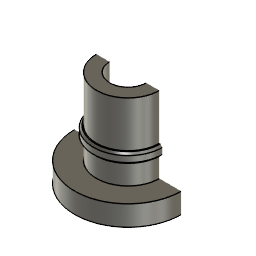
Alfa 147 Handle Saddle V3 - 3.6mm (Autodesk Fusion 360 design; units mm, degrees)
Autodesk Fusion 360 part; units mm, degrees
sketch "Sketch1" plane through (0, 0, 0) normal (0, 0, 1) x (1, 0, 0)
  circle A0 centre (0, 0) radius 5.25
  circle A1 centre (0, 0) radius 3.1
  circle A2 centre (0, 0) radius 1.8
  circle A3 centre (0, 0) radius 3.4
  circle A4 centre (0, 0) radius 1.5
  dimension "d1" = 10.5
  dimension "d2" = 6.2
  dimension "d3" = 3.6
  dimension "d21" = 0.3
  dimension "d22" = 0.3
  constraint coincident A0.centre A1.centre
  constraint concentric A0 A2
  constraint concentric A2 A3
  constraint concentric A1 A4
  measures "d1" diameter of A0
  measures "d2" diameter of A1
  measures "d3" diameter of A2
  measures "d21" distance of A2 A4
  measures "d22" distance of A1 A3
extrude "Extrude1" add sketch "Sketch1" along normal blind 9.5 contours A1
extrude "Extrude2" add sketch "Sketch1" along normal blind 2 contours A0 | A3
extrude "Extrude3" add sketch "Sketch1" along normal blind 4 and the other way blind -5 contours A3
chamfer "Chamfer1" distance 0.2 angle 45 2 edges at (-3.1699, -1.2295, 4) (-3.1699, -1.2295, 5)
chamfer "Chamfer2" distance 0.5 angle 45 1 edges at (-1.6782, 0.6509, 0)
extrude "Extrude4" add sketch "Sketch1" along normal blind 5 and the other way blind -4 contours A2
chamfer "Chamfer3" distance 0.2 angle 45 2 edges at (-1.3985, 0.5424, 5) (-1.3985, 0.5424, 4)
equation "d2 = OuterRadius"
equation "d3 = InnerRadius"
equation "d21 = NotchThickness"
equation "d22 = NotchThickness"
equation "InnerRadius = 3.6 mm"
equation "OuterRadius = 6.2 mm"
equation "NotchThickness = 0.30 mm"
